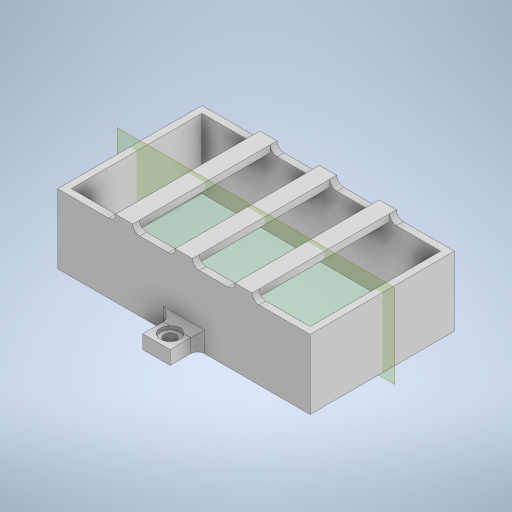
# Autodesk Inventor part: battery_holder
Saved by Autodesk Inventor 2024.2 (Build 282272000, 272)
## iProperties
Created: 2024-03-06
Part Number: battery_holder
Material: Generic
Document SubType Name: Modeling
Designer: crow
Density: 1 g/cm^3
Appearance: Default
Author: crow
## iProperties of the stored document battery_holder_3DPrint.ipt
Created: 2024-03-06
Part Number: battery_holder_3DPrint
Material: Generic
Document SubType Name: Modeling
Designer: crow
Density: 1 g/cm^3
Appearance: Default
Author: crow
Autodesk Inventor part; units mm, degrees
ref_plane "YZ Plane" through (0, 0, 0) normal (1, 0, 0) x (0, 1, 0)
ref_plane "XZ Plane" through (0, 0, 0) normal (0, 1, 0) x (-1, 0, 0)
ref_plane "XY Plane" through (0, 0, 0) normal (0, 0, 1) x (1, 0, 0)
sketch "Sketch1" plane through (0, 0, 0) normal (0, 1, 0) x (-1, 0, 0)
  line L0 (-47.2438, -20.2959) -> (22.2562, -20.2959)
  line L1 (22.2562, -20.2959) -> (22.2562, 17.7041)
  line L2 (22.2562, 17.7041) -> (-47.2438, 17.7041)
  line L3 (-47.2438, 17.7041) -> (-47.2438, -20.2959)
  line L4 (-49.2438, -22.2959) -> (24.2562, -22.2959)
  line L5 (24.2562, -22.2959) -> (24.2562, 19.7041)
  line L6 (24.2562, 19.7041) -> (-49.2438, 19.7041)
  line L7 (-49.2438, 19.7041) -> (-49.2438, -22.2959)
  line L8 (-12.4938, 0) -> (-12.4938, -4.6169) construction
  line L9 (-12.4938, 17.7041) -> (-12.4938, -20.2959) construction
  line L10 (24.2562, -2.25) -> (24.2562, 2.25)
  line L11 (-49.2438, 2.25) -> (-49.2438, -2.25)
  line L12 (-8.4938, -30.2959) -> (-16.4938, -30.2959)
  line L13 (-16.4938, -30.2959) -> (-16.4938, -20.2959)
  line L14 (-16.4938, -20.2959) -> (-8.4938, -20.2959)
  line L15 (-8.4938, -20.2959) -> (-8.4938, -30.2959)
  line L16 (-12.4938, -30.2959) -> (-12.4938, -20.2959) construction
  line L17 (22.2562, -1.2959) -> (-47.2438, -1.2959) construction
  point P0 (0, 0)
  point P1 (-12.4938, -26.2959)
  point P2 (-12.4938, -22.2959)
  dimension "d0" = 69.5
  dimension "d1" = 38
  dimension "d2" = 2
  dimension "d3" = 2
  dimension "d4" = 2
  dimension "d5" = 2
  dimension "d10" = 4.5
  dimension "d34" = 4
  dimension "d36" = 8
  dimension "d38" = 4
  constraints: 36 end point, 7 midpoint, 6 parallel, 3 horizontal, 3 perpendicular, 1 collinear, 1 point on line, 1 vertical
  measures "d0" distance of L2.end L1.end
  measures "d1" distance of L1.end L0.end
  measures "d2" distance between parallel lines of L1 L5
  measures "d3" distance between parallel lines of L2 L6
  measures "d4" distance between parallel lines of L3 L7
  measures "d5" distance between parallel lines of L0 L4
  measures "d10" distance of L11.start L11.end
  measures "d34" distance of point (-12.494, -26.296) point (-12.494, -22.296)
  measures "d36" distance of L13.end L14.end
  measures "d38" distance from line of L12 point (-12.494, -26.296)
extrude "Extrusion1" add sketch "Sketch1" along normal blind 20.2 contours L0 L13 L4 L7 L6 L5 L15 L1 L2 L3 | L0 L15 L4 L13
extrude "Extrusion2" add sketch "Sketch1" along normal blind 4 contours L0 L15 L4 L13 | L4 L15 L12 L13
sketch "Sketch2" plane through (0, 20.2, 0) normal (0, 1, 0) x (1, 0, 0)
  line L0 (49.2438, 22.2959) -> (-24.2562, 22.2959) projected
  line L1 (-24.2562, -19.7041) -> (49.2438, -19.7041) projected
  line L2 (-7.3812, 22.2959) -> (-2.3812, 22.2959)
  line L3 (-2.3812, 22.2959) -> (-2.3812, -19.7041)
  line L4 (-2.3812, -19.7041) -> (-7.3812, -19.7041)
  line L5 (-7.3812, -19.7041) -> (-7.3812, 22.2959)
  line L6 (-22.2562, -17.7041) -> (-22.2562, 20.2959) projected
  line L7 (9.9938, 22.2959) -> (14.9938, 22.2959)
  line L8 (14.9938, 22.2959) -> (14.9938, -19.7041)
  line L9 (14.9938, -19.7041) -> (9.9938, -19.7041)
  line L10 (9.9938, -19.7041) -> (9.9938, 22.2959)
  line L11 (27.3688, 22.2959) -> (32.3688, 22.2959)
  line L12 (32.3688, 22.2959) -> (32.3688, -19.7041)
  line L13 (32.3688, -19.7041) -> (27.3688, -19.7041)
  line L14 (27.3688, -19.7041) -> (27.3688, 22.2959)
  line L15 (12.4938, 22.2959) -> (12.4938, -19.7041) construction
  line L16 (29.8688, 22.2959) -> (29.8688, -19.7041) construction
  point P0 (0, 0)
  point P1 (14.9938, 22.2959)
  dimension "d22" = 5
  dimension "d24" = 5
  dimension "d26" = 5
  dimension "d28" = 2.5
  dimension "d29" = 12.375
  dimension "d30" = 17.375
  dimension "d31" = 12.375
  constraints: 28 end point, 8 point on line, 6 parallel, 4 perpendicular, 3 horizontal, 2 midpoint
  measures "d22" distance of L3.end L4.end
  measures "d24" distance of L8.end L9.end
  measures "d26" distance of L12.end L13.end
  measures "d28" distance between parallel lines of L15 L10
  measures "d29" distance between parallel lines of L14 L8
  measures "d30" distance between parallel lines of L16 L15
  measures "d31" distance between parallel lines of L10 L3
extrude "Extrusion3" add sketch "Sketch2" along normal blind 2 contours L12 L1 L14 L0 | L8 L1 L10 L0 | L3 L1 L5 L0
sketch "Sketch3" plane through (0, 4, 0) normal (0, 1, 0) x (1, 0, 0)
  line L0 (16.4938, 22.2959) -> (16.4938, 30.2959) construction
  line L1 (16.4938, 26.2959) -> (8.4938, 26.2959) construction
  line L2 (8.4938, 30.2959) -> (8.4938, 22.2959) construction
  line L3 (16.4938, 30.2959) -> (8.4938, 30.2959) construction
  line L4 (12.4938, 30.2959) -> (12.4938, 22.2959) construction
  line L5 (16.4938, 22.2959) -> (8.4938, 22.2959) construction
  point P0 (0, 0)
  point P1 (12.4938, 26.2959)
  constraints: 5 midpoint, 4 end point
hole "Hole2" at (12.4938, 4, -26.2959) direction (0, -1, 0) diameter 3.4 depth 6 counterbore diameter 5.62 counterbore depth 1 clearance for "Countersunk Flat Head Screw ISO 2009/7046" size "M3" standard "ISO"
fillet "Fillet1" radius 2 2 edges at (8.4938, 2, -22.2959) (16.4938, 2, -22.2959)
fillet "Fillet2" radius 2 1 edges at (12.4938, 4, -22.2959)
ref_plane "Work Plane1" through (-24.2562, 0, -1.2959) normal (0, 0, -1) x (-1, 0, 0)
mirror "Mirror1" about plane through (-24.2562, 0, -1.2959) normal (0, 0, -1) of "Fillet2", "Fillet1", "Extrusion2", "Hole2"
fillet "Fillet3" radius 2 12 edges at (32.3688, 20.2, 18.7041) (27.3688, 20.2, 18.7041) (14.9938, 20.2, 18.7041) (9.9938, 20.2, 18.7041) (-7.3812, 20.2, 18.7041) (-2.3812, 20.2, 18.7041) (-2.3812, 20.2, -21.2959) (14.9938, 20.2, -21.2959) (32.3688, 20.2, -21.2959) (27.3688, 20.2, -21.2959) (9.9938, 20.2, -21.2959) (-7.3812, 20.2, -21.2959)
equation "\"d31\" = d29"
body "Solid1"
